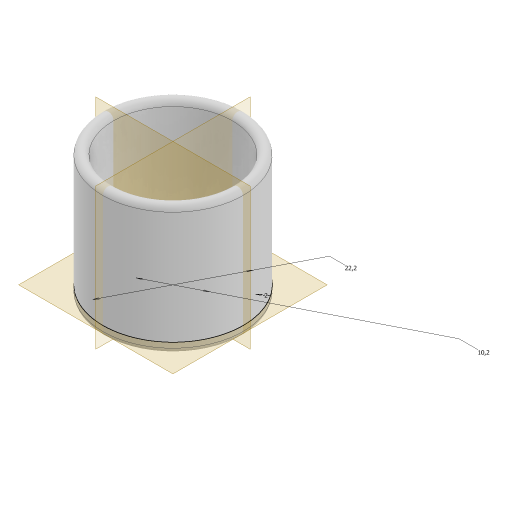
# Autodesk Inventor part: Стакан для крепления ходовой гайки
Saved by Autodesk Inventor 2023.2 (Build 272271030, 271C)
## iProperties
Created: 2025-04-10
Part Number: Стакан для крепления ходовой гайки
Material: Типовые
Document SubType Name: Modeling
Designer: Коноваленко
Density: 1 g/cm^3
Appearance: По умолчанию
Author: Коноваленко
Autodesk Inventor part; units mm, degrees
sketch "Эскиз1" plane through (0, 0, 0) normal (0, 1, 0) x (-1, 0, 0)
  circle A0 centre (0, 0) radius 11.1
  circle A1 centre (0, 0) radius 13.1
  circle A2 centre (0, 0) radius 5.1
  dimension "d0" = 22.2
  dimension "d1" = 2
  dimension "d2" = 10.2
  constraints: 3 centre point, 3 coincident
  measures "d0" diameter of A0
  measures "d1" radial gap between concentric circles of A1 A0
  measures "d2" diameter of A2
extrude "Выдавливание1" add sketch "Эскиз1" along normal blind 22 contours A1
extrude "Выдавливание2" add sketch "Эскиз1" against normal blind 2 contours A0 | A1
fillet "Сопряжение1" radius 1 2 edges at (13.1, 22, 0) (11.1, 22, 0)
fillet "Сопряжение2" radius 1 1 edges at (13.1, -2, 0)
